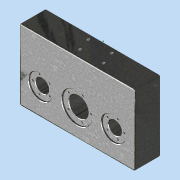
# Autodesk Inventor part: mitte
Saved by Autodesk Inventor 2021 (Build 250183000, 183)
## iProperties
Created: 2024-03-14
Part Number: mitte
Material: Generic
Document SubType Name: Modeling
Designer: Nokia
Density: 1 g/cm^3
Appearance: Steel Galvanized
Mass: 2261.83 g
Surface Area: 1621.77 cm^2
Volume: 2261.83 cm^3
Author: Nokia
Autodesk Inventor part; units mm, degrees
ref_plane "YZ Plane" through (0, 0, 0) normal (1, 0, 0) x (0, 1, 0)
ref_plane "XZ Plane" through (0, 0, 0) normal (0, 1, 0) x (-1, 0, 0)
ref_plane "XY Plane" through (0, 0, 0) normal (0, 0, 1) x (1, 0, 0)
sketch "Sketch1" plane through (0, 0, 0) normal (0, 0, 1) x (1, 0, 0)
  line L0 (130, 80) -> (130, -80)
  line L1 (130, -80) -> (-130, -80)
  line L2 (-130, -80) -> (-130, 80)
  line L3 (-130, 80) -> (130, 80)
  point P0 (0, 0)
  dimension "d2" = 260
  dimension "d3" = 160
  constraints: 8 end point, 3 perpendicular
  measures "d2" distance of L0.end L1.end
  measures "d3" distance of L1.end L2.end
extrude "Extrusion1" add sketch "Sketch1" along normal blind 60
sketch "Sketch2" plane through (0, 0, 60) normal (0, 0, 1) x (1, 0, 0)
  circle A0 centre (0, -20) radius 22
  line L0 (130, 80) -> (-130, 80) projected
  circle A1 centre (0, -20) radius 34
  circle A2 centre (27.998, -20.3313) radius 3
  circle A3 centre (8.9669, 6.5253) radius 3
  circle A4 centre (-22.4562, -3.2751) radius 3
  circle A5 centre (-22.8456, -36.1888) radius 3
  circle A6 centre (8.3368, -46.7301) radius 3
  line L1 (130, -80) -> (130, 80) projected
  dimension "d10" = 100
  dimension "d76" = 44
  dimension "d77" = 68
  dimension "d82" = 6
  dimension "d85" = 360
  dimension "d145" = 28
  dimension "d146" = 130
  constraints: 7 centre point, 1 coincident, 11 other
  measures "d10" distance from line of L0 A0.centre
  measures "d76" diameter of A0
  measures "d77" diameter of A1
  measures "d82" diameter of A2
  measures "d145" distance of A0.centre A2.centre
  measures "d146" distance from line of L1 A0.centre
extrude "Extrusion2" cut sketch "Sketch2" against normal blind 60 contours A0
sketch "Sketch3" plane through (-130, 80, 0) normal (0, 1, 0) x (1, 0, 0)
  line L0 (130, 0) -> (140.9191, -30)
  line L1 (260, 0) -> (0, 0) projected
  line L2 (0, -60) -> (260, -60) projected
  line L3 (73.8413, -60) -> (206.9951, -60)
  line L4 (0, 0) -> (0, -60) projected
  line L5 (0, 0) -> (0, 58.141)
  line L6 (114.7929, 41.7812) -> (67.8083, 24.6802)
  line L7 (103.3956, 0) -> (108.5259, -14.0954)
  circle A0 centre (108.5259, -14.0954) radius 5
  line L8 (108.5259, -14.0954) -> (118.7865, -42.2862)
  circle A1 centre (118.7865, -42.2862) radius 5
  line L9 (130, 0) -> (130, -19.9546)
  line L10 (108, -60) -> (108, 0) projected
  line L11 (152, -60) -> (152, 0) projected
  line L12 (114.7929, 41.7812) -> (138.2852, 50.3317)
  line L13 (108.5259, -14.0954) -> (161.7347, -14.0954)
  line L14 (118.7865, -42.2862) -> (171.9954, -42.2862)
  circle A2 centre (161.7347, -14.0954) radius 5
  circle A3 centre (171.9954, -42.2862) radius 5
  dimension "d20" = 70
  dimension "d39" = 50
  dimension "d40" = 70
  dimension "d49" = 10
  dimension "d57" = 15
  dimension "d65" = 30
  dimension "d66" = 10
  dimension "d67" = 20
  dimension "d68" = 20
  dimension "d71" = 25
  dimension "d74" = 10
  dimension "d75" = 10
  constraints: 20 end point, 4 centre point, 4 coincident, 4 point on line, 2 perpendicular, 1 vertical
  measures "d20" angle of L1 L0
  measures "d39" distance of L6.start L6.end
  measures "d40" angle of L6 L5
  measures "d49" diameter of A0
  measures "d57" distance of L7.start L7.end
  measures "d65" distance of L7.end L8.end
  measures "d66" diameter of A1
  measures "d67" angle of L9 L0
  measures "d68" angle of L10 L8
  measures "d71" distance of L6.start L12.end
  measures "d74" diameter of A2
  measures "d75" diameter of A3
hole "Hole5" at (-21.4741, 80, 14.0954) at (-11.2135, 80, 42.2862) at (31.7347, 80, 14.0954) at (41.9954, 80, 42.2862) direction (0, -1, 0) diameter 6.647 depth 43 tip angle 118 thread size "M8x1.25" class "6H" standard "ISO Metric profile"
extrude "Extrusion3" cut sketch "Sketch2" against normal blind 4 contours A1 | A2 | A3 | A4 | A5 | A6
sketch "Sketch4" plane through (0, 0, 0) normal (0, 0, -1) x (-1, 0, 0)
  circle A0 centre (0, -20) radius 34 projected
  circle A1 centre (0, -20) radius 34
  circle A2 centre (0, -20) radius 22
  line L0 (130, 80) -> (-130, 80)
  circle A3 centre (0, -20) radius 34
  circle A4 centre (28, -20) radius 3
  circle A5 centre (8.6525, 6.6296) radius 3
  circle A6 centre (-22.6525, -3.542) radius 3
  circle A7 centre (-22.6525, -36.458) radius 3
  circle A8 centre (8.6525, -46.6296) radius 3
  point P0 (0, 0)
  dimension "d89" = 100
  dimension "d90" = 44
  dimension "d91" = 68
  dimension "d92" = 6
  dimension "d93" = 360
  dimension "d147" = 12
  dimension "d148" = 28
  constraints: 8 centre point, 2 coincident, 2 end point, 11 other
  measures "d89" distance from line of L0 A2.centre
  measures "d90" diameter of A2
  measures "d91" diameter of A3
  measures "d92" diameter of A4
  measures "d147" radial gap between concentric circles of A0 A2
  measures "d148" distance of A1.centre A4.centre
extrude "Extrusion4" cut sketch "Sketch4" against normal blind 4 contours A0 | A2 | A4 | A5 | A6 | A7 | A8
hole "Hole6" at (-8.6525, -46.6296, 0) at (22.6525, -36.458, 0) at (22.6525, -3.542, 0) at (-8.6525, 6.6296, 0) at (-28, -20, 0) direction (0, 0, 1) diameter 4.134 depth 28 tip angle 118 thread size "M5x0.8" class "6H" standard "ISO Metric profile"
hole "Hole7" at (8.9669, 6.5253, 60) at (27.998, -20.3313, 60) at (8.3368, -46.7301, 60) at (-22.8456, -36.1888, 60) at (-22.4562, -3.2751, 60) direction (0, 0, -1) diameter 4.134 depth 28 tip angle 118 thread size "M5x0.8" class "6H" standard "ISO Metric profile"
sketch "Sketch5" plane through (0, 0, 60) normal (0, 0, 1) x (1, 0, 0)
  line L0 (130, -80) -> (130, 80) projected
  circle A0 centre (-82, -20) radius 15
  circle A1 centre (82, -20) radius 15
  line L1 (-130, 80) -> (-130, -80) projected
  circle A2 centre (-82, -20) radius 27
  circle A3 centre (0, -20) radius 22 projected
  line L2 (0, 0) -> (0, -20)
  circle A4 centre (82, -20) radius 27
  dimension "d108" = 30
  dimension "d112" = 48
  dimension "d113" = 48
  dimension "d114" = 30
  dimension "d117" = 54
  constraints: 4 centre point, 2 end point, 1 coincident, 1 symmetric about line, 1 vertical, 1 other
  measures "d108" diameter of A0
  measures "d112" distance from line of L1 A0.centre
  measures "d113" distance from line of L0 A1.centre
  measures "d114" diameter of A1
  measures "d117" diameter of A2
extrude "Extrusion6" cut sketch "Sketch5" against normal through all contours A0 | A1
extrude "Extrusion7" cut sketch "Sketch5" against normal blind 4 contours A2 | A4
sketch "Sketch7" plane through (0, 0, 0) normal (0, 0, -1) x (-1, 0, 0)
  circle A0 centre (-82, -20) radius 13
  circle A1 centre (82, -20) radius 13
  circle A2 centre (-82, -20) radius 27
  circle A3 centre (0, -20) radius 22
  line L0 (0, 0) -> (0, -20)
  circle A4 centre (82, -20) radius 27
  point P0 (130, -80)
  point P1 (-130, -80)
  dimension "d120" = 26
  dimension "d121" = 26
  dimension "d122" = 54
  constraints: 5 centre point, 2 end point, 1 coincident, 1 symmetric about line, 1 vertical, 1 other
  measures "d120" diameter of A0
  measures "d121" diameter of A1
  measures "d122" diameter of A2
extrude "Extrusion8" cut sketch "Sketch7" against normal blind 4 contours A2 | A4
sketch "Sketch8" plane through (-82, -20, 4) normal (0, 0, -1) x (-1, 0, 0)
  circle A0 centre (0, 0) radius 15 projected
  circle A1 centre (21, 0) radius 2.5
  circle A2 centre (6.4894, 19.9722) radius 2.5
  circle A3 centre (-16.9894, 12.3435) radius 2.5
  circle A4 centre (-16.9894, -12.3435) radius 2.5
  circle A5 centre (6.4894, -19.9722) radius 2.5
  circle A6 centre (-82, 0) radius 22 projected
  line L0 (-82, 20) -> (-82, 0)
  circle A7 centre (-185, 0) radius 2.5
  circle A8 centre (-170.4894, 19.9722) radius 2.5
  circle A9 centre (-147.0106, 12.3435) radius 2.5
  circle A10 centre (-147.0106, -12.3435) radius 2.5
  circle A11 centre (-170.4894, -19.9722) radius 2.5
  dimension "d126" = 5
  dimension "d129" = 360
  dimension "d143" = 0
  dimension "d144" = 21
  constraints: 10 centre point, 5 symmetric about line, 2 end point, 1 coincident, 1 vertical, 16 other
  measures "d126" diameter of A1
  measures "d143" vertical distance of A0.centre point (21, 0)
  measures "d144" distance of A0.centre point (21, 0)
sketch "Sketch9" plane through (82, -20, 56) normal (0, 0, 1) x (1, 0, 0)
  circle A0 centre (0, 0) radius 13
  circle A1 centre (21, 0) radius 2.5
  circle A2 centre (6.4894, 19.9722) radius 2.5
  circle A3 centre (-16.9894, 12.3435) radius 2.5
  circle A4 centre (-16.9894, -12.3435) radius 2.5
  circle A5 centre (6.4894, -19.9722) radius 2.5
  circle A6 centre (-82, 0) radius 22
  line L0 (-82, 20) -> (-82, 0)
  circle A7 centre (-185, 0) radius 2.5
  circle A8 centre (-170.4894, -19.9722) radius 2.5
  circle A9 centre (-170.4894, 19.9722) radius 2.5
  circle A10 centre (-147.0106, 12.3435) radius 2.5
  circle A11 centre (-147.0106, -12.3435) radius 2.5
  dimension "d134" = 5
  dimension "d135" = 360
  dimension "d151" = 21
  constraints: 12 centre point, 5 symmetric about line, 2 end point, 1 vertical, 16 other
  measures "d134" diameter of A1
  measures "d151" distance of A0.centre A1.centre
hole "Hole8" at (-103, -20, 4) at (-88.4894, -39.9722, 4) at (-65.0106, -32.3435, 4) at (-65.0106, -7.6565, 4) at (-88.4894, -0.0278, 4) at (65.0106, -7.6565, 4) at (88.4894, -0.0278, 4) at (103, -20, 4) at (88.4894, -39.9722, 4) at (65.0106, -32.3435, 4) direction (0, 0, 1) diameter 4.134 depth 24 tip angle 118 thread size "M5x0.8" class "6H" standard "ISO Metric profile"
hole "Hole9" at (88.4894, -0.0278, 56) at (103, -20, 56) at (88.4894, -39.9722, 56) at (65.0106, -32.3435, 56) at (65.0106, -7.6565, 56) at (-65.0106, -32.3435, 56) at (-65.0106, -7.6565, 56) at (-88.4894, -0.0278, 56) at (-103, -20, 56) at (-88.4894, -39.9722, 56) direction (0, 0, -1) diameter 4.134 depth 24 tip angle 118 thread size "M5x0.8" class "6H" standard "ISO Metric profile"
fillet "Fillet1" radius 4 12 edges at (0, 80, 60) (0, 80, 0) (0, -80, 0) (0, -80, 60) (130, 0, 60) (130, 0, 0) (-130, 0, 0) (-130, 0, 60) (-130, 80, 30) (130, 80, 30) (130, -80, 30) (-130, -80, 30)
chamfer "Chamfer1" distance 0.5 angle 45 34 edges at (-11.2135, 80, 38.9627) (41.9954, 80, 38.9627) (31.7347, 80, 10.7719) (-21.4741, 80, 10.7719) (-88.4894, 2.0392, 56) (-65.0106, -5.5895, 56) (-65.0106, -30.2765, 56) (-88.4894, -37.9052, 56) (-103, -17.933, 56) (-22.8456, -34.1218, 56) (-22.4562, -1.2081, 56) (8.9669, 8.5923, 56) (27.998, -18.2643, 56) (8.3368, -44.6631, 56) (65.0106, -30.2765, 56) (88.4894, -37.9052, 56) (103, -17.933, 56) (88.4894, 2.0392, 56) (65.0106, -5.5895, 56) (88.4894, -2.0948, 4) (103, -22.067, 4) (88.4894, -42.0392, 4) (65.0106, -34.4105, 4) (65.0106, -9.7235, 4) (22.6525, -5.609, 4) (-8.6525, 4.5626, 4) (-28, -22.067, 4) (-8.6525, -48.6966, 4) (22.6525, -38.525, 4) (-65.0106, -34.4105, 4) (-65.0106, -9.7235, 4) (-88.4894, -2.0948, 4) (-103, -22.067, 4) (-88.4894, -42.0392, 4)
chamfer "Chamfer2" distance 1 angle 45 12 edges at (109, -20, 0) (67, -20, 4) (-22, -20, 4) (34, -20, 0) (-55, -20, 0) (-97, -20, 4) (-34, -20, 60) (-22, -20, 56) (67, -20, 56) (55, -20, 60) (-109, -20, 60) (-97, -20, 56)
body "Solid1"
